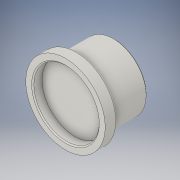
# Autodesk Inventor part: Loer die 2 center
Saved by Autodesk Inventor 2017 (Build 210142000, 142)
## iProperties
Created: 2017-04-13
Part Number: Loer die 2 center
Material: Steel
Document SubType Name: Modeling
Designer: rbibb
Mass: 370.353 g
Surface Area: 104.61 cm^2
Volume: 47.1788 cm^3
Density: 7.85 g/cm^3
Appearance: Steel
Author: rbibb
Autodesk Inventor part; units mm, degrees
ref_plane "YZ Plane" through (0, 0, 0) normal (1, 0, 0) x (0, 1, 0)
ref_plane "XZ Plane" through (0, 0, 0) normal (0, 1, 0) x (-1, 0, 0)
ref_plane "XY Plane" through (0, 0, 0) normal (0, 0, 1) x (1, 0, 0)
sketch "Sketch1" plane through (0, 0, 0) normal (1, 0, 0) x (0, 1, 0)
  line L0 (-3.195, -4.0211) -> (-3.195, -25.8564)
  line L1 (-3.195, -25.8564) -> (19.03, -25.8564)
  line L2 (19.03, -25.8564) -> (19.03, -0.4564)
  line L3 (19.03, -0.4564) -> (23.7925, -0.4564)
  line L4 (23.7925, -0.4564) -> (23.7925, 0)
  line L5 (19.03, 1.1311) -> (-3.195, 1.1311)
  line L6 (-3.195, 1.1311) -> (-3.195, -4.0211)
  line L7 (19.03, 1.1311) -> (19.03, 7.4811)
  line L8 (19.03, 7.4811) -> (23.7925, 7.4811)
  line L9 (23.7925, 7.4811) -> (23.7925, 0)
  dimension "d1" = 4.7625
  dimension "d2" = 7.9375
  dimension "d3" = 6.35
  dimension "d5" = 26.9875
  dimension "d6" = 22.225
  constraints: 20 end point, 4 parallel, 1 horizontal, 1 perpendicular, 1 point on line
  measures "d1" distance of L7.end L8.end
  measures "d2" distance of L3.end L8.end
  measures "d3" distance of L5.start L7.end
  measures "d5" horizontal distance of L8.end L5.end
  measures "d6" distance of L0.end L1.end
revolve "Revolution1" add sketch "Sketch1" angle 360 about axis through (0, -3.195, -4.0211) along (0, 0, -1)
sketch "Sketch2" plane through (0, -3.195, -25.8564) normal (0, 0, -1) x (-1, 0, 0)
  point P0 (0, 3.195)
sketch "Sketch3" plane through (0, -3.195, -25.8564) normal (0, 0, -1) x (-1, 0, 0)
  point P0 (0, 3.195)
  point P1 (0, 0)
hole "Hole1" at (0, -3.195, -25.8564) direction (0, 0, 1) diameter 4.9784 depth 19.05 tip angle 118 countersink diameter 9.525 countersink angle 82 thread size "1/4-20 UNC" class "2B" standard "ANSI Unified Screw Threads"
chamfer "Chamfer1" distance 0.762 angle 45 1 edges at (0, -25.42, 7.4811) measured on face at (-3.9258, 21.7283, 7.4811)
chamfer "Chamfer2" distance 0.762 angle 45 1 edges at (0, -25.42, -25.8564) measured on face at (-2.1528, 12.9477, -25.8564)
fillet "Fillet1" radius 0.7874 1 edges at (0, -30.1825, -0.4564)
body "Solid1"
